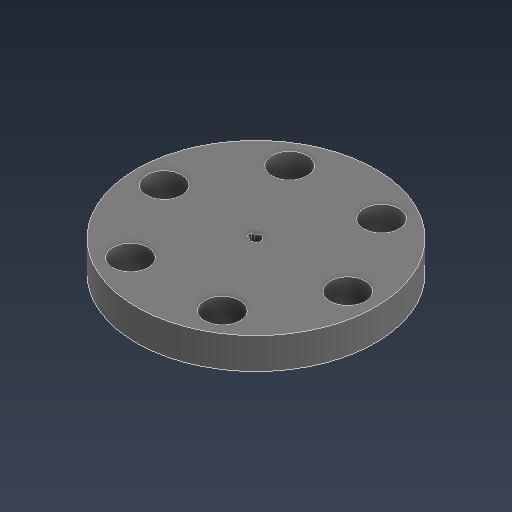
# Autodesk Inventor part: ballInletWheel
Saved by Autodesk Inventor 2021.4 (Build 254397000, 397)
## iProperties
Created: 2021-11-23
Part Number: ballInletWheel
Material: Generic
Document SubType Name: Modeling
Designer: jo_ki
Density: 1 g/cm^3
Appearance: Gray
Author: jo_ki
Autodesk Inventor part; units mm, degrees
ref_plane "YZ Plane" through (0, 0, 0) normal (1, 0, 0) x (0, 1, 0)
ref_plane "XZ Plane" through (0, 0, 0) normal (0, 1, 0) x (-1, 0, 0)
ref_plane "XY Plane" through (0, 0, 0) normal (0, 0, 1) x (1, 0, 0)
derived "Mastersketch.ipt"
sketch "Sketch1" plane through (0, 0, 0) normal (0, 1, 0) x (-1, 0, 0)
  circle A0 centre (0, 0) radius 118.9738
  circle A1 centre (0, 0) radius 5
  line L0 (7, 2.5) -> (0, 2.5)
  line L1 (0, 2.5) -> (0, -2.5)
  line L2 (0, -2.5) -> (7, -2.5)
  line L3 (7, -2.5) -> (7, 2.5)
  line L4 (7, 2.5) -> (0, -2.5) construction
  line L5 (0, 2.5) -> (7, -2.5) construction
  line L6 (0, -166.8083) -> (0, 166.8083) projected
  line L7 (166.8083, 0) -> (-166.8083, 0) projected
  circle A2 centre (0, 0) radius 7
  point P0 (3.5, 0)
  point P1 (5, 0)
  point P2 (5, 0)
  point P3 (4.3301, 2.5)
  point P4 (4.3301, -2.5)
  point P5 (7, 0)
  point P6 (6.5383, 2.5)
  point P7 (6.5383, -2.5)
  dimension "d2" = 10
  dimension "d1" = 237.9477
  dimension "d3" = 2
  dimension "d4" = 5
  constraints: 12 end point, 4 coincident, 4 midpoint, 2 parallel, 1 centre point, 1 collinear, 1 horizontal, 1 perpendicular, 1 point on line, 7 other
  measures "d1" diameter of A0
  measures "d3" distance from line of L3 point (5, 0)
  measures "d4" distance between parallel lines of L0 L2
extrude "Extrusion1" add sketch "Sketch1" along normal mid plane 31 contours L7 L3 L0 A2 L6 A0 | A0 L6 A2 L2 L3 L7 | L6 A2 L7 A0 | A0 L7 A2 L6 | A2 L0 L3 | L3 L2 A2 | A2 L0 A1 L6 | L6 A1 L7 A2 | A2 L7 A1 L6 | L6 A1 L2 A2
sketch "Sketch2" plane through (0, 15.5, 0) normal (0, 1, 0) x (1, 0, 0)
  circle A0 centre (-91.4738, 0) radius 17.5
  line L0 (-166.7734, 0) -> (166.5984, 0) projected
  circle A1 centre (0, 0) radius 118.9738 projected
  point P0 (-118.9738, 0)
  point P1 (-108.9738, 0)
  dimension "d7" = 35
  dimension "d9" = 10
  constraints: 3 point on line, 2 horizontal alignment, 3 other
  measures "d9" distance of point (-108.974, 0) point (-118.974, 0)
sketch "Sketch3" plane through (0, 0, 0) normal (0, 0, 1) x (1, 0, 0)
  line L0 (118.9738, 15.5) -> (-118.9738, 15.5) projected
  line L1 (-91.4738, 15.5) -> (-86.0077, -15.5)
  line L2 (-118.9738, -15.5) -> (118.9738, -15.5) projected
  point P0 (0, 0)
  dimension "d10" = 80
  constraints: 3 point on line, 2 end point
  measures "d10" angle of L0 L1
sweep "Sweep1" cut profiles "Sketch2" path "Sketch3" path curves L1 contours L0 A0 | A0 L0
pattern_circular "Circular Pattern1" count 6 over 360 about axis through (0, -10, 0) along (0, 1, 0) of "Sweep1"
equation "\"d2\" = ballInletWheelDriveShaftAxle_diameter"
equation "\"d1\" = ballInletWheel_diameter"
equation "\"d5\" = ballInletWheel_thickness"
equation "\"d7\" = ball_size + 2 * ball_rollTolerance"
equation "\"d9\" = ballInletWheel_margin"
equation "\"ballInletWheelDriveShaftAxle_diameter\" = 10"
equation "\"ballInletWheel_diameter\" = 237.947682"
equation "\"ballInletWheel_thickness\" = 31"
equation "\"ball_size\" = 33"
equation "\"ball_rollTolerance\" = 1"
equation "\"ballInletWheel_margin\" = 10"
body "Solid1"
